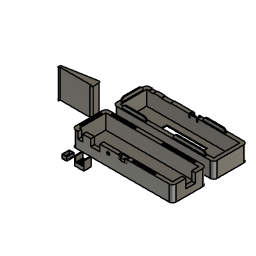
Weather station v1.1 (Autodesk Fusion 360 design; units mm, degrees)
Autodesk Fusion 360 part; units mm, degrees
sketch "Sketch1" plane through (0, 0, 0) normal (0, 0, 1) x (1, 0, 0)
  line L0 (-80, 20.5981) -> (83.75, 20.5981)
  line L1 (83.75, 20.5981) -> (83.75, -25.5019)
  line L2 (83.75, -25.5019) -> (-80, -25.5019)
  line L3 (-80, -25.5019) -> (-80, 20.5981)
  line L4 (-86.5, -32.0019) -> (-86.5, 27.0981)
  line L5 (-86.5, 27.0981) -> (90.25, 27.0981)
  line L6 (90.25, 27.0981) -> (90.25, -32.0019)
  line L7 (90.25, -32.0019) -> (-86.5, -32.0019)
  dimension "d1" = 163.75
  dimension "d2" = 46.1
  dimension "d11" = -6.5
  constraint horizontal L0
  constraint vertical L1
  constraint horizontal L2
  constraint vertical L3
  measures "d1" distance of L0.start L0.end
  measures "d2" distance of L0.start L2.end
extrude "Extrude3" add sketch "Sketch1" along normal blind 1.25 contours L0 L1 L2 L3 makes body 1
extrude "Extrude4" add sketch "Sketch1" along normal blind 55 bodies 1
fillet "Fillet2" radius 6 4 edges at (90.25, -32.0019, 27.5) (90.25, 27.0981, 27.5) (-86.5, -32.0019, 27.5) (-86.5, 27.0981, 27.5) on bodies 1
sketch "Sketch5" plane through (0, 0, 0) normal (0, 0, -1) x (1, 0, 0)
  arc A0 (-86.5, -21.0981) -> (-80.5, -27.0981) centre (-80.5, -21.0981) ccw
  line L0 (-80.5, -27.0981) -> (84.25, -27.0981)
  arc A1 (84.25, -27.0981) -> (90.25, -21.0981) centre (84.25, -21.0981) ccw
  line L1 (90.25, -21.0981) -> (90.25, 26.0019)
  arc A2 (90.25, 26.0019) -> (84.25, 32.0019) centre (84.25, 26.0019) ccw
  line L2 (84.25, 32.0019) -> (-80.5, 32.0019)
  arc A3 (-80.5, 32.0019) -> (-86.5, 26.0019) centre (-80.5, 26.0019) ccw
  line L3 (-86.5, 26.0019) -> (-86.5, -21.0981)
move_body "Move1" bodies 1 to x (1, 0, 0) y (0, 1, 0) z (0, 0, 1) at (-1.875, 2.4519, 0)
sketch "Sketch8" plane through (0, 0, 55) normal (0, 0, 1) x (-1, 0, 0)
  line L0 (-81.875, 23.05) -> (81.875, 23.05)
  line L1 (81.875, 23.05) -> (81.875, -23.05)
  line L2 (81.875, -23.05) -> (-81.875, -23.05)
  line L3 (-81.875, -23.05) -> (-81.875, 23.05)
  arc A0 (82.375, -29.55) -> (88.375, -23.55) centre (82.375, -23.55) ccw
  line L4 (88.375, -23.55) -> (88.375, 23.55)
  arc A1 (88.375, 23.55) -> (82.375, 29.55) centre (82.375, 23.55) ccw
  line L5 (82.375, 29.55) -> (-82.375, 29.55)
  arc A2 (-82.375, 29.55) -> (-88.375, 23.55) centre (-82.375, 23.55) ccw
  line L6 (-88.375, 23.55) -> (-88.375, -23.55)
  arc A3 (-88.375, -23.55) -> (-82.375, -29.55) centre (-82.375, -23.55) ccw
  line L7 (-82.375, -29.55) -> (82.375, -29.55)
  line L8 (39.6596, 23.05) -> (55.7404, 23.05)
  line L9 (55.7404, 23.05) -> (55.7404, 29.55)
  line L10 (55.7404, 29.55) -> (39.6596, 29.55)
  line L11 (39.6596, 29.55) -> (39.6596, 23.05)
  line L12 (69.8395, 23.05) -> (78.1187, 23.05)
  line L13 (78.1187, 23.05) -> (78.1187, 29.55)
  line L14 (78.1187, 29.55) -> (69.8395, 29.55)
  line L15 (69.8395, 29.55) -> (69.8395, 23.05)
  line L16 (-81.875, 6.2908) -> (-88.375, 6.2908)
  line L17 (-88.375, 6.2908) -> (-88.375, -10.6862)
  line L18 (-88.375, -10.6862) -> (-81.875, -10.6862)
  line L19 (-81.875, -10.6862) -> (-81.875, 6.2908)
  constraint horizontal L8
  constraint vertical L9
  constraint horizontal L10
  constraint vertical L11
  constraint coincident L5 L9.end
  constraint coincident L0 L8.start
  constraint horizontal L12
  constraint vertical L13
  constraint horizontal L14
  constraint vertical L15
  constraint coincident L5 L13.end
  constraint coincident L0 L12.start
  constraint horizontal L16
  constraint vertical L17
  constraint horizontal L18
  constraint vertical L19
  constraint coincident L6 L17.end
  constraint coincident L3 L16.start
sketch "Sketch9" plane through (0, 0, 55) normal (0, 0, 1) x (-1, 0, 0)
  line L0 (-81.875, -23.05) -> (-81.875, 23.05)
  line L1 (-81.875, 23.05) -> (81.875, 23.05)
  line L2 (82.375, 29.55) -> (-82.375, 29.55)
  arc A0 (-82.375, 29.55) -> (-88.375, 23.55) centre (-82.375, 23.55) ccw
  line L3 (-88.375, 23.55) -> (-88.375, -23.55)
  line L4 (5.8, 23.1) -> (7.8, 23.1)
  line L5 (7.8, 23.1) -> (7.8, 25.1)
  line L6 (7.8, 25.1) -> (5.8, 25.1)
  line L7 (5.8, 25.1) -> (5.8, 23.1)
  line L8 (-5.6999, 23.05) -> (-7.6999, 23.05)
  line L9 (-7.6999, 23.05) -> (-7.6999, 25.05)
  line L10 (-7.6999, 25.05) -> (-5.6999, 25.05)
  line L11 (-5.6999, 25.05) -> (-5.6999, 23.05)
  line L12 (7.8, 25.1) -> (-7.7, 25.1)
  line L13 (-7.7, 25.1) -> (-7.7, 28.6)
  line L14 (-7.7, 28.6) -> (7.8, 28.6)
  line L15 (7.8, 28.6) -> (7.8, 25.1)
  line L16 (-4, 28.6) -> (4, 28.6)
  line L17 (4, 28.6) -> (4, 30.6)
  line L18 (4, 30.6) -> (-4, 30.6)
  line L19 (-4, 30.6) -> (-4, 28.6)
  line L20 (81.875, 23.05) -> (81.875, -23.05)
  line L21 (81.875, -23.05) -> (-81.875, -23.05)
  arc A1 (82.375, -29.55) -> (88.375, -23.55) centre (82.375, -23.55) ccw
  line L22 (88.375, -23.55) -> (88.375, 23.55)
  arc A2 (88.375, 23.55) -> (82.375, 29.55) centre (82.375, 23.55) ccw
  arc A3 (-88.375, -23.55) -> (-82.375, -29.55) centre (-82.375, -23.55) ccw
  line L23 (-82.375, -29.55) -> (82.375, -29.55)
  dimension "d37" = 11.5
  dimension "d38" = 2
  dimension "d39" = 2
  dimension "d40" = 2
  dimension "d41" = 2
  dimension "d42" = 15.5
  dimension "d43" = 3.5
  dimension "d44" = 8
  dimension "d45" = 2
  constraint horizontal L4
  constraint vertical L5
  constraint horizontal L6
  constraint vertical L7
  constraint horizontal L8
  constraint vertical L9
  constraint horizontal L10
  constraint vertical L11
  constraint coincident L1 L8.end
  constraint horizontal L12
  constraint vertical L13
  constraint horizontal L14
  constraint vertical L15
  constraint horizontal L16
  constraint vertical L17
  constraint horizontal L18
  constraint vertical L19
  constraint coincident L14 L16.start
  measures "d37" distance of L8.start L4.start
  measures "d38" distance of L4.start L4.end
  measures "d39" distance of L4.start L6.end
  measures "d40" distance of L8.start L8.end
  measures "d41" distance of L8.start L10.end
  measures "d42" distance of L5.end L12.end
  measures "d43" distance of L5.end L14.end
  measures "d44" distance of L16.start L16.end
  measures "d45" distance of L16.start L18.end
extrude "Extrude10" cut sketch "Sketch9" against normal blind 13 from surface at -21.5 contours L1 L8 L9 L10 L11 | L2 L14 L16 L17 L19 | L6 L12 L13 L14 L15 L16 | L4 L5 L6 L7 L12 bodies 1
extrude "Extrude11" cut sketch "Sketch8" against normal blind 13 from surface at -26.5 contours L0 L5 L8 L9 L10 L11 | L0 L5 L12 L13 L14 L15 bodies 1
extrude "Extrude12" cut sketch "Sketch8" against normal blind 16 from surface at -27.5 contours L3 L6 L16 L17 L18 L19 bodies 1
sketch "Sketch11" plane through (0, 23.05, 0) normal (0, -1, 0) x (1, 0, 0)
  line L0 (-81.875, 1.25) -> (81.875, 1.25)
  line L1 (81.875, 1.25) -> (81.875, 55)
  line L2 (81.875, 55) -> (-81.875, 55)
  line L3 (-81.875, 55) -> (-81.875, 1.25)
  line L4 (-81.875, 55) -> (81.875, 55)
  line L5 (81.875, 55) -> (81.875, 53.25)
  line L6 (81.875, 53.25) -> (-81.875, 53.25)
  line L7 (-81.875, 53.25) -> (-81.875, 55)
  dimension "d59" = 1.75
  constraint horizontal L4
  constraint vertical L5
  constraint horizontal L6
  constraint vertical L7
  constraint coincident L2.end L3.start
  measures "d59" distance of L2.end L6.end
extrude "Extrude13" add sketch "Sketch11" along normal blind 47 contours L1 L2 L3 L4 L5 L6 L7 bodies 1
sketch "Sketch13" plane through (0, 0, 55) normal (0, 0, 1) x (-1, 0, 0)
  arc A0 (82.375, -29.55) -> (88.375, -23.55) centre (82.375, -23.55) ccw
  line L0 (88.375, -23.55) -> (88.375, 23.55)
  arc A1 (88.375, 23.55) -> (82.375, 29.55) centre (82.375, 23.55) ccw
  line L1 (82.375, 29.55) -> (-82.375, 29.55)
  arc A2 (-82.375, 29.55) -> (-88.375, 23.55) centre (-82.375, 23.55) ccw
  line L2 (-88.375, 23.55) -> (-88.375, -23.55)
  arc A3 (-88.375, -23.55) -> (-82.375, -29.55) centre (-82.375, -23.55) ccw
  line L3 (-82.375, -29.55) -> (82.375, -29.55)
  line L4 (35.625, 12.075) -> (-35.625, 12.075)
  line L5 (-35.625, 12.075) -> (-35.625, -12.075)
  line L6 (-35.625, -12.075) -> (35.625, -12.075)
  line L7 (35.625, -12.075) -> (35.625, 12.075)
  line L8 (35.625, 12.075) -> (-35.625, -12.075) construction
  line L9 (-35.625, 12.075) -> (35.625, -12.075) construction
  dimension "d62" = 71.25
  dimension "d63" = 24.15
  constraint horizontal L4
  constraint perpendicular L4 L5
  constraint parallel L4 L6
  constraint parallel L5 L7
  constraint coincident L8 origin
  constraint coincident L9 origin
  measures "d62" distance of L5.end L6.end
  measures "d63" distance of L4.end L5.end
extrude "Extrude14" cut sketch "Sketch13" against normal blind 5 contours L4 L5 L6 L7 bodies 1
sketch "Sketch14" plane through (0, -29.55, 0) normal (0, -1, 0) x (1, 0, 0)
  line L0 (-39.6596, 28.5) -> (-39.6596, 15.5)
  line L1 (-39.6596, 15.5) -> (-55.7404, 15.5)
  line L2 (-55.7404, 15.5) -> (-55.7404, 28.5)
  line L3 (-55.7404, 28.5) -> (-39.6596, 28.5)
  line L4 (-69.8395, 28.5) -> (-69.8395, 15.5)
  line L5 (-69.8395, 15.5) -> (-78.1187, 15.5)
  line L6 (-78.1187, 15.5) -> (-78.1187, 28.5)
  line L7 (-78.1187, 28.5) -> (-69.8395, 28.5)
  line L8 (-4, 20.5) -> (-4, 33.5)
  line L9 (-4, 33.5) -> (4, 33.5)
  line L10 (4, 33.5) -> (4, 20.5)
  line L11 (4, 20.5) -> (-4, 20.5)
  line L12 (-82.375, 55) -> (-82.375, 0)
  line L13 (-82.375, 0) -> (82.375, 0)
  line L14 (82.375, 0) -> (82.375, 55)
  line L15 (82.375, 55) -> (-82.375, 55)
  circle A0 centre (-26.6402, 20.4154) radius 0.375
  circle A1 centre (-23.6402, 20.4154) radius 0.375
  dimension "d66" = 0.75
  dimension "d67" = 0.75
  measures "d66" diameter of A0
  measures "d67" diameter of A1
extrude "Extrude15" cut sketch "Sketch14" against normal blind 7 contours A0 | A1 bodies 1
sketch "Sketch15" plane through (0, -29.55, 0) normal (0, -1, 0) x (1, 0, 0)
  circle A0 centre (-23.6402, 20.4154) radius 0.375
  circle A1 centre (-26.6402, 20.4154) radius 0.375
  line L0 (-39.6596, 28.5) -> (-39.6596, 15.5)
  line L1 (-39.6596, 15.5) -> (-55.7404, 15.5)
  line L2 (-55.7404, 15.5) -> (-55.7404, 28.5)
  line L3 (-55.7404, 28.5) -> (-39.6596, 28.5)
  line L4 (-69.8395, 28.5) -> (-69.8395, 15.5)
  line L5 (-69.8395, 15.5) -> (-78.1187, 15.5)
  line L6 (-78.1187, 15.5) -> (-78.1187, 28.5)
  line L7 (-78.1187, 28.5) -> (-69.8395, 28.5)
  line L8 (-4, 20.5) -> (-4, 33.5)
  line L9 (-4, 33.5) -> (4, 33.5)
  line L10 (4, 33.5) -> (4, 20.5)
  line L11 (4, 20.5) -> (-4, 20.5)
  line L12 (-82.375, 55) -> (-82.375, 0)
  line L13 (-82.375, 0) -> (82.375, 0)
  line L14 (82.375, 0) -> (82.375, 55)
  line L15 (82.375, 55) -> (-82.375, 55)
  line L16 (-26.6402, 20.4154) -> (-23.6402, 20.4154)
  line L17 (-25.1402, 18.1654) -> (-26.6402, 18.1654)
  line L18 (-25.1402, 18.1654) -> (-23.6402, 18.1654)
  line L19 (-25.1402, 22.6654) -> (-26.6402, 22.6654)
  line L20 (-25.1402, 22.6654) -> (-23.6402, 22.6654)
  line L21 (-23.6402, 20.4154) -> (-22.4402, 20.4154)
  arc A2 (-23.6402, 18.1654) -> (-23.6402, 22.6654) centre (-25.1496, 20.4154) ccw
  line L22 (-26.6402, 20.4154) -> (-27.8402, 20.4154)
  arc A3 (-26.6402, 22.6654) -> (-26.6402, 18.1654) centre (-25.1308, 20.4154) ccw
  dimension "d72" = 1.5
  dimension "d73" = 1.5
  dimension "d74" = 1.5
  dimension "d75" = 1.5
  dimension "d76" = 1.2
  dimension "d77" = 1.2
  constraint coincident A1.centre L16.start
  constraint coincident A0.centre L16.end
  constraint parallel L16 L21
  constraint coincident L21.end A2
  constraint parallel L16 L22
  constraint coincident L22.end A3
  measures "d72" distance of L17.start L17.end
  measures "d73" distance of L17.start L18.end
  measures "d74" distance of L19.start L19.end
  measures "d75" distance of L19.start L20.end
  measures "d76" distance of A0.centre L21.end
  measures "d77" distance of A1.centre L22.end
extrude "Extrude16" cut sketch "Sketch15" against normal blind 2 contours A0 A1 L16 L17 L18 L21 A2 L22 A3 | A0 A1 L16 L19 L20 L21 A2 L22 A3 bodies 1
sketch "Sketch16" plane through (0, 0, 0) normal (0, 0, 1) x (1, 0, 0)
  line L0 (110, 30) -> (185, 30)
  line L1 (185, 30) -> (185, -30)
  line L2 (185, -30) -> (110, -30)
  line L3 (110, -30) -> (110, 30)
  constraint horizontal L0
  constraint vertical L1
  constraint horizontal L2
  constraint vertical L3
extrude "Extrude17" add sketch "Sketch16" along normal blind 27.5 separate body makes body 2
split "Split1" by plane through (0, 0, 27.5) normal (0, 0, 1) bodies 1 makes body 3 at (70.7917, 4.025, 55)
sketch "Sketch18" plane through (0, 0, 27.5) normal (0, 0, 1) x (-1, 0, 0)
  line L0 (75, -27.5712) -> (75, -25.3712)
  line L1 (75, -25.3712) -> (32.2569, -25.3712)
  line L2 (32.2569, -25.3712) -> (32.2569, -27.5712)
  line L3 (32.2569, -27.5712) -> (75, -27.5712)
  line L4 (85, -19) -> (86, -19)
  line L5 (86, -19) -> (86, 19)
  line L6 (86, 19) -> (83.8, 19)
  line L7 (83.8, 19) -> (83.8, -19)
  line L8 (83.8, -19) -> (85, -19)
  line L9 (-15, 27) -> (-55, 27)
  line L10 (-55, 27) -> (-55, 24.8)
  line L11 (-55, 24.8) -> (-15, 24.8)
  line L12 (-15, 24.8) -> (-15, 27)
  line L13 (-14.7553, -27.3712) -> (-72.1053, -27.3712)
  line L14 (-72.1053, -27.3712) -> (-72.1053, -25.1712)
  line L15 (-72.1053, -25.1712) -> (-14.7553, -25.1712)
  line L16 (-14.7553, -25.1712) -> (-14.7553, -27.3712)
  dimension "d82" = 2.2
  dimension "d104" = 2.2
  dimension "d105" = 2.2
  dimension "d106" = 2.2
  constraint vertical L0
  constraint perpendicular L0 L1
  constraint perpendicular L1 L2
  constraint perpendicular L2 L3
  constraint horizontal L9
  constraint vertical L10
  constraint horizontal L11
  constraint vertical L12
  constraint horizontal L13
  constraint vertical L14
  constraint horizontal L15
  constraint vertical L16
  measures "d82" distance of L1.end L2.end
  measures "d104" distance of L9.start L11.end
  measures "d105" distance of L13.start L15.end
  measures "d106" distance of L5.end L6.end
sketch "Sketch31" plane through (0, -29.55, 0) normal (0, -1, 0) x (1, 0, 0)
  line L0 (-55.7404, 27.5) -> (-69.8395, 27.5)
  line L1 (-69.8395, 27.5) -> (-69.8395, 15.5)
  line L2 (-69.8395, 15.5) -> (-78.1187, 15.5)
  line L3 (-78.1187, 15.5) -> (-78.1187, 27.5)
  line L4 (-78.1187, 27.5) -> (-82.375, 27.5)
  line L5 (-82.375, 27.5) -> (-82.375, 0)
  line L6 (-82.375, 0) -> (82.375, 0)
  line L7 (82.375, 0) -> (82.375, 27.5)
  line L8 (82.375, 27.5) -> (4, 27.5)
  line L9 (4, 27.5) -> (4, 20.5)
  line L10 (4, 20.5) -> (-4, 20.5)
  line L11 (-4, 20.5) -> (-4, 27.5)
  line L12 (-4, 27.5) -> (-39.6596, 27.5)
  line L13 (-39.6596, 27.5) -> (-39.6596, 15.5)
  line L14 (-39.6596, 15.5) -> (-55.7404, 15.5)
  line L15 (-55.7404, 15.5) -> (-55.7404, 27.5)
  arc A0 (-26.6402, 22.6654) -> (-26.6402, 18.1654) centre (-25.1308, 20.4154) ccw
  line L16 (-26.6402, 22.6654) -> (-23.6402, 22.6654)
  arc A1 (-23.6402, 18.1654) -> (-23.6402, 22.6654) centre (-25.1496, 20.4154) ccw
  line L17 (-23.6402, 18.1654) -> (-26.6402, 18.1654)
  line L18 (-69.8895, 15.55) -> (-69.8895, 28.45)
  line L19 (-69.8895, 28.45) -> (-78.0687, 28.45)
  line L20 (-78.0687, 28.45) -> (-78.0687, 15.55)
  line L21 (-78.0687, 15.55) -> (-69.8895, 15.55)
  line L22 (-39.71, 15.55) -> (-39.71, 28.45)
  line L23 (-39.71, 28.45) -> (-55.6904, 28.45)
  line L24 (-55.6904, 28.45) -> (-55.6904, 15.55)
  line L25 (-55.6904, 15.55) -> (-39.71, 15.55)
extrude "Extrude35" cut sketch "Sketch18" against normal blind 15 bodies 1
sketch "Sketch30" plane through (0, 0, 27.5) normal (0, 0, 1) x (-1, 0, 0)
  line L0 (86, -18.9875) -> (86, 18.9893)
  line L1 (85, -18.9875) -> (86, -18.9875)
  line L2 (83.8, 18.9893) -> (83.8, -18.9875)
  line L3 (32.2569, -27.5712) -> (75, -27.5712)
  line L4 (-55, 27) -> (-55, 24.8)
  line L5 (-55, 24.8) -> (-15, 24.8)
  line L6 (-15, 24.8) -> (-15, 27)
  line L7 (-72.1053, -27.3712) -> (-72.1053, -25.1712)
  line L8 (86, 18.9893) -> (83.8, 18.9893)
  line L9 (75, -27.5712) -> (75, -25.3712)
  line L10 (-15, 27) -> (-55, 27)
  line L11 (-72.1053, -25.1712) -> (-14.7553, -25.1712)
  line L12 (83.8, -18.9875) -> (85, -18.9875)
  line L13 (75, -25.3712) -> (32.2569, -25.3712)
  line L14 (-14.7553, -25.1712) -> (-14.7553, -27.3712)
  line L15 (-14.7553, -27.3712) -> (-72.1053, -27.3712)
  line L16 (32.2569, -25.3712) -> (32.2569, -27.5712)
  line L17 (-15.125, 26.875) -> (-54.875, 26.875)
  line L18 (-54.875, 26.875) -> (-54.875, 24.925)
  line L19 (-54.875, 24.925) -> (-15.125, 24.925)
  line L20 (-15.125, 24.925) -> (-15.125, 26.875)
  line L21 (-71.9803, -25.2962) -> (-14.8803, -25.2962)
  line L22 (-14.8803, -25.2962) -> (-14.8803, -27.2462)
  line L23 (-14.8803, -27.2462) -> (-71.9803, -27.2462)
  line L24 (-71.9803, -27.2462) -> (-71.9803, -25.2962)
  line L25 (74.875, -25.4962) -> (32.3819, -25.4962)
  line L26 (32.3819, -25.4962) -> (32.3819, -27.4462)
  line L27 (32.3819, -27.4462) -> (74.875, -27.4462)
  line L28 (74.875, -27.4462) -> (74.875, -25.4962)
  line L29 (83.925, 18.8643) -> (83.925, -18.8625)
  line L30 (83.925, -18.8625) -> (85, -18.8625)
  line L31 (85, -18.8625) -> (85.875, -18.8625)
  line L32 (85.875, -18.8625) -> (85.875, 18.8643)
  line L33 (85.875, 18.8643) -> (83.925, 18.8643)
  line L34 (75, -25.3712) -> (75, -27.5712)
  line L35 (75, -27.5712) -> (32.2569, -27.5712)
  line L36 (32.2569, -27.5712) -> (32.2569, -25.3712)
  line L37 (32.2569, -25.3712) -> (75, -25.3712)
  line L38 (-72.1053, -27.3712) -> (-72.1053, -25.1712)
  line L39 (-72.1053, -25.1712) -> (-14.7553, -25.1712)
  line L40 (-14.7553, -25.1712) -> (-14.7553, -27.3712)
  line L41 (-14.7553, -27.3712) -> (-72.1053, -27.3712)
  line L42 (86, 19) -> (86, -19)
  line L43 (86, -19) -> (83.8, -19)
  line L44 (83.8, -19) -> (83.8, 19)
  line L45 (83.8, 19) -> (86, 19)
  arc A0 (-88.375, -23.55) -> (-82.375, -29.55) centre (-82.375, -23.55) ccw
  line L46 (-82.375, -29.55) -> (82.375, -29.55)
  arc A1 (82.375, -29.55) -> (88.375, -23.55) centre (82.375, -23.55) ccw
  line L47 (88.375, -23.55) -> (88.375, 23.55)
  arc A2 (88.375, 23.55) -> (82.375, 29.55) centre (82.375, 23.55) ccw
  line L48 (82.375, 29.55) -> (78.1187, 29.55)
  line L49 (78.1187, 29.55) -> (78.1187, 23.05)
  line L50 (78.1187, 23.05) -> (81.875, 23.05)
  line L51 (81.875, 23.05) -> (81.875, -23.05)
  line L52 (81.875, -23.05) -> (-81.875, -23.05)
  line L53 (-81.875, -23.05) -> (-81.875, -10.6862)
  line L54 (-81.875, -10.6862) -> (-88.375, -10.6862)
  line L55 (-88.375, -10.6862) -> (-88.375, -23.55)
  dimension "d163" = 2.2
  dimension "d164" = 2.2
  dimension "d165" = 2.2
  dimension "d166" = 2.2
  dimension "d167" = -0.125
  dimension "d168" = 0.125
  dimension "d169" = -0.125
  dimension "d170" = -0.125
  constraint vertical L9
  constraint perpendicular L9 L13
  constraint perpendicular L13 L16
  constraint perpendicular L3 L16
  constraint horizontal L10
  constraint vertical L4
  constraint horizontal L5
  constraint vertical L6
  constraint horizontal L15
  constraint vertical L7
  constraint horizontal L11
  constraint vertical L14
  measures "d163" distance of L13.end L3.start
  measures "d164" distance of L5.end L6.end
  measures "d165" distance of L14.end L11.end
  measures "d166" distance of L0.end L2.start
extrude "Extrude40" add sketch "Sketch30" against normal blind 6 contours L17 L18 L19 L20 | L21 L22 L23 L24 | L25 L26 L27 L28 | L29 L30 L31 L32 L33 bodies 3
fillet "Fillet7" radius 6 8 edges at (15.125, -25.9, 21.5) (54.875, -25.9, 21.5) (71.9803, 26.2712, 21.5) (14.8803, 26.2712, 21.5) (-32.3819, 26.4712, 21.5) (-74.875, 26.4712, 21.5) (-84.9, -18.8643, 21.5) (-84.9, 18.8625, 21.5) on bodies 3
sketch "Sketch37" plane through (-88.375, 0, 0) normal (-1, 0, 0) x (0, -1, 0)
  line L0 (-23.55, 27.5) -> (23.55, 27.5)
  line L1 (23.55, 27.5) -> (23.55, 55)
  line L2 (23.55, 55) -> (-23.55, 55)
  line L3 (-23.55, 55) -> (-23.55, 27.5)
  line L4 (-32.55, 55) -> (-32.55, 0)
  line L5 (-29.55, 0) -> (-29.55, 55)
  line L6 (-26.55, 58) -> (-32.55, 58)
  line L7 (-32.55, 58) -> (-32.55, 55)
  line L8 (-26.55, -3) -> (-32.55, -3)
  line L9 (-32.55, -3) -> (-32.55, 0)
  line L10 (-32.55, 58) -> (-42.777, 0)
  line L11 (-32.55, 58) -> (26.3447, 58) construction
  line L12 (-42.777, 0) -> (-32.55, 0)
  line L13 (-42.777, 0) -> (-32.55, 0)
  line L14 (-32.55, 0) -> (-32.55, -3)
  line L15 (-32.55, -3) -> (-42.777, -3)
  line L16 (-42.777, -3) -> (-42.777, 0)
  line L17 (-32.55, 55.075) -> (-26.55, 55.075)
  line L18 (-26.55, 55.075) -> (-26.55, 58)
  line L19 (-29.55, 55) -> (-29.55, 55.075)
  line L20 (-32.55, -0.08) -> (-26.55, -0.08)
  line L21 (-26.55, -0.08) -> (-26.55, -3)
  line L22 (-29.55, 0) -> (-29.55, -0.08)
  dimension "d215" = 3
  dimension "d217" = 3
  dimension "d219" = 3
  dimension "d220" = 100
  constraint vertical L4
  constraint vertical L5
  constraint horizontal L6
  constraint vertical L7
  constraint horizontal L8
  constraint vertical L9
  constraint horizontal L11
  constraint perpendicular L9 L12
  constraint horizontal L13
  constraint vertical L14
  constraint horizontal L15
  constraint vertical L16
  constraint perpendicular L6 L18
  constraint midpoint L17 L19.end
  constraint perpendicular L17 L19
  constraint perpendicular L8 L21
  constraint midpoint L20 L22.end
  constraint perpendicular L20 L22
  constraint coincident L9 L20.start
  constraint perpendicular L9 L20
  measures "d215" distance of L5.end L4.start
  measures "d217" distance of L4.start L6.end
  measures "d219" distance of L4.end L8.end
  measures "d220" angle of L10 L11
extrude "Extrude56" add sketch "Sketch37" against normal blind 50 separate body contours L4 L5 L7 L9 L14 L17 L19 L20 L22 | L4 L7 L10 L12 L13 | L9 L12 L13 L14 L15 L16 | L6 L7 L17 L18 | L8 L9 L14 L20 L21 makes body 4
fillet "Fillet10" radius 3 4 edges at (-63.375, 32.55, 58) (-63.375, 26.55, 58) (-63.375, 42.777, -3) (-63.375, 26.55, -3) on bodies 4
move_body "Move17" bodies 3 to x (1, 0, 0) y (0, -1, 0) z (0, 0, -1) at (0, -5.7601, 110)
move_body "Move18" bodies 3 to x (1, 0, 0) y (0, 1, 0) z (0, 0, 1) at (0, 17.8351, -55)
move_body "Move19" bodies 3 to x (1, 0, 0) y (0, 1, 0) z (0, 0, 1) at (0, 60, 0)
extrude "Extrude42" add sketch "Sketch31" against normal blind 6.5 separate body contours L18 L19 L20 L21 | L22 L23 L24 L25 makes body 5 at (-50.3636, -29.55, 19.85) makes body 6 at (-72.6159, -29.55, 19.85)
move_body "Move23" bodies 5 6 to x (1, 0, 0) y (0, 0, 1) z (0, -1, 0) at (0, -47.1661, 48.9339)
move_body "Move24" bodies 5 6 to x (1, 0, 0) y (0, 1, 0) z (0, 0, 1) at (47.7002, 69.1661, -19.3839)
move_body "Move25" bodies 5 6 to x (1, 0, 0) y (0, 1, 0) z (0, 0, 1) at (-48, -51, 0)
sketch "Sketch32" plane through (0, 0, 6.5) normal (0, 0, 1) x (-1, 0, 0)
  line L0 (40.0098, 44.55) -> (55.9902, 44.55)
  line L1 (55.9902, 44.55) -> (55.9902, 57.45)
  line L2 (55.9902, 57.45) -> (40.0098, 57.45)
  line L3 (40.0098, 57.45) -> (40.0098, 44.55)
  line L4 (54.5, 56) -> (41.5, 56)
  line L5 (41.5, 56) -> (41.5, 54)
  line L6 (41.5, 54) -> (54.5, 54)
  line L7 (54.5, 54) -> (54.5, 56)
  line L8 (54.5, 46) -> (41.5, 46)
  line L9 (41.5, 46) -> (41.5, 48)
  line L10 (41.5, 48) -> (54.5, 48)
  line L11 (54.5, 48) -> (54.5, 46)
  line L12 (41.5, 52) -> (54.5, 52)
  line L13 (54.5, 52) -> (54.5, 50)
  line L14 (54.5, 50) -> (41.5, 50)
  line L15 (41.5, 50) -> (41.5, 52)
  constraint horizontal L4
  constraint vertical L5
  constraint horizontal L6
  constraint vertical L7
  constraint horizontal L8
  constraint vertical L9
  constraint horizontal L10
  constraint vertical L11
  constraint horizontal L12
  constraint vertical L13
  constraint horizontal L14
  constraint vertical L15
extrude "Extrude43" cut sketch "Sketch32" against normal blind 7 contours L4 L5 L6 L7 | L8 L9 L10 L11 | L12 L13 L14 L15 bodies 5
sketch "Sketch33" plane through (0, 0, 6.5) normal (0, 0, 1) x (-1, 0, 0)
  line L0 (70.1894, 44.55) -> (78.3686, 44.55)
  line L1 (78.3686, 44.55) -> (78.3686, 57.45)
  line L2 (78.3686, 57.45) -> (70.1894, 57.45)
  line L3 (70.1894, 57.45) -> (70.1894, 44.55)
  line L4 (77.5, 56.5) -> (71, 56.5)
  line L5 (71, 56.5) -> (71, 45.5)
  line L6 (71, 45.5) -> (77.5, 45.5)
  line L7 (77.5, 45.5) -> (77.5, 56.5)
  constraint horizontal L4
  constraint vertical L5
  constraint horizontal L6
  constraint vertical L7
extrude "Extrude44" cut sketch "Sketch33" against normal blind 4.5 contours L4 L5 L6 L7 bodies 6
sketch "Sketch34" plane through (0, 0, 6.5) normal (0, 0, 1) x (-1, 0, 0)
  line L0 (41.5, 56) -> (54.5, 56)
  line L1 (54.5, 56) -> (54.5, 54)
  line L2 (54.5, 54) -> (41.5, 54)
  line L3 (41.5, 54) -> (41.5, 56)
  line L4 (54.5, 52) -> (54.5, 50)
  line L5 (54.5, 50) -> (41.5, 50)
  line L6 (41.5, 50) -> (41.5, 52)
  line L7 (41.5, 52) -> (54.5, 52)
  line L8 (41.5, 46) -> (41.5, 48)
  line L9 (41.5, 48) -> (54.5, 48)
  line L10 (54.5, 48) -> (54.5, 46)
  line L11 (54.5, 46) -> (41.5, 46)
  line L12 (40.0098, 44.55) -> (55.9902, 44.55)
  line L13 (55.9902, 44.55) -> (55.9902, 57.45)
  line L14 (55.9902, 57.45) -> (40.0098, 57.45)
  line L15 (40.0098, 57.45) -> (40.0098, 44.55)
  line L16 (55.9902, 44.55) -> (54.5, 44.55)
  line L17 (54.5, 44.55) -> (54.5, 57.45)
  line L18 (54.5, 57.45) -> (55.9902, 57.45)
  line L19 (55.9902, 57.45) -> (55.9902, 44.55)
  line L20 (40.0098, 44.55) -> (41.5, 44.55)
  line L21 (41.5, 44.55) -> (41.5, 57.45)
  line L22 (41.5, 57.45) -> (40.0098, 57.45)
  line L23 (40.0098, 57.45) -> (40.0098, 44.55)
  constraint horizontal L16
  constraint vertical L17
  constraint horizontal L18
  constraint vertical L19
  constraint coincident L14 L17.end
  constraint coincident L12.end L13.start
  constraint horizontal L20
  constraint vertical L21
  constraint horizontal L22
  constraint vertical L23
  constraint coincident L14 L21.end
  constraint coincident L12.start L15.end
extrude "Extrude45" add sketch "Sketch34" along normal blind 9 contours L3 L6 L8 L12 L14 L15 L20 L21 L22 L23 | L1 L4 L10 L12 L13 L14 L16 L17 L18 L19 bodies 5
extrude "Extrude47" add 1 faces at (-45.8333, -57.45, 2.1667) along direction (0, -1, 0) blind 0.05 on bodies 5 bodies 5
extrude "Extrude48" add 1 faces at (-72.9158, -57.45, 2.1667) along direction (0, -1, 0) blind 0.05 on bodies 6 bodies 6
extrude "Extrude49" add 1 faces at (-70.1894, -53.1834, 2.1667) along direction (1, 0, 0) blind 0.05 on bodies 6 bodies 6
extrude "Extrude50" add 1 faces at (-40.0098, -53.1833, 10.3333) along direction (1, 0, 0) blind 0.05 on bodies 5 bodies 5
extrude "Extrude51" add 1 faces at (-45.8167, -44.55, 2.1667) along direction (0, 1, 0) blind 0.05 on bodies 5 bodies 5
extrude "Extrude52" add 1 faces at (-72.8824, -44.55, 4.3333) along direction (0, 1, 0) blind 0.05 on bodies 6 bodies 6
extrude "Extrude53" add 1 faces at (-78.3686, -53.1667, 2.1667) along direction (-1, 0, 0) blind 0.05 on bodies 6 bodies 6
extrude "Extrude54" add 1 faces at (-55.9902, -53.1667, 10.3333) along direction (-1, 0, 0) blind 0.05 on bodies 5 bodies 5
move_body "Move27" bodies 4 to x (1, 0, 0) y (0, 1, 0) z (0, 0, 1) at (-70, 0, 0)
move_body "Move28" bodies 4 to x (0, 0, 1) y (0, 1, 0) z (-1, 0, 0) at (-105.8775, 0, 160.8725)
move_body "Move29" bodies 4 to x (1, 0, 0) y (0, 1, 0) z (0, 0, 1) at (-8.0158, 0.4105, -2.4975)
extrude "Extrude57" cut 1 faces at (-6.4667, -23.1, 25.1667) along direction (0, 1, 0) blind 1 on bodies 1 bodies 1
extrude "Extrude58" cut 1 faces at (7.0332, 97.125, 23.5) along direction (0, 1, 0) blind 1 on bodies 3 bodies 3
extrude "Extrude59" cut 1 faces at (-6.4667, 95.175, 23.5) along direction (0, -1, 0) blind 1 on bodies 3 bodies 3
extrude "Extrude60" cut 1 faces at (7.0332, -25.05, 25.1667) along direction (0, -1, 0) blind 1 on bodies 1 bodies 1
move_body "Move30" [rolled back]
hidden bodies 2
named bodies: "Bottom half", "Splitting body (Hidden)", "Top half", "Sensor cover", "LED cover", "Tilt bracket"
